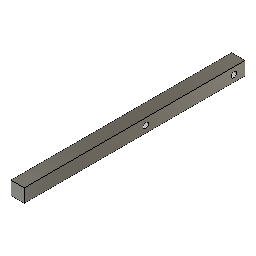
module_bolt (Autodesk Fusion 360 design; units mm, degrees)
Autodesk Fusion 360 part; units mm, degrees
sketch "Skizze1" plane through (0, 0, 0) normal (0, 1, 0) x (1, 0, 0)
  line L0 (0, 0) -> (6, 0)
  line L1 (6, 0) -> (6, -6)
  line L2 (6, -6) -> (0, -6)
  line L3 (0, -6) -> (0, 0)
  dimension "d1" = 6
  dimension "d2" = 6
  constraint horizontal L0
  constraint vertical L1
  constraint horizontal L2
  constraint vertical L3
  constraint coincident L0.start L3.end
  measures "d1" distance of L0.start L0.end
  measures "d2" distance of L0.end L1.end
extrude "Extrusion1" add sketch "Skizze1" along normal blind 100
sketch "Skizze2" plane through (6, 0, 0) normal (1, 0, 0) x (0, 1, 0)
  line L0 (0, 6) -> (0, 0)
  line L1 (0, 0) -> (100, 0)
  line L2 (100, 0) -> (100, 6)
  line L3 (100, 6) -> (0, 6)
  point P0 (95, 3)
  point P1 (55, 3)
  dimension "d5" = 3
  dimension "d6" = 3
  dimension "d7" = 5
  dimension "d8" = 45
  measures "d5" distance of L1 P1
  measures "d6" distance of L1 P0
  measures "d7" distance of L2 P0
  measures "d8" distance of L2 P1
hole "Bohrung1" at (6, 95, 3) at (6, 55, 3) direction (-1, 0, 0) diameter 2.529 depth 30 tip angle 118
thread "Gewinde1" "ISO Metric profile 3.0 M3x0.5 6H"
